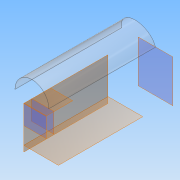
# Autodesk Inventor part: Top_Guard 1
Saved by Autodesk Inventor 2018.1 (Build 221171000, 171)
## iProperties
Created: 2019-03-23
Part Number: Top_Guard 1
Material: PMMA Plastic
Document SubType Name: Modeling
Designer: James
Density: 1.188 g/cm^3
Appearance: Polycarbonate - Clear
Author: James
Autodesk Inventor part; units mm, degrees
ref_plane "YZ Plane" through (0, 0, 0) normal (1, 0, 0) x (0, 1, 0)
ref_plane "XZ Plane" through (0, 0, 0) normal (0, 1, 0) x (-1, 0, 0)
ref_plane "XY Plane" through (0, 0, 0) normal (0, 0, 1) x (1, 0, 0)
derived "Top_Skeleton.ipt"
ref_plane "Work Plane1" through (0, 0, 0) normal (0, 0, 1) x (1, 0, 0)
ref_plane "Work Plane2" through (0, 0, 0) normal (0, 1, 0) x (-1, 0, 0)
ref_plane "Work Plane3" through (0, 0, 0) normal (1, 0, 0) x (0, 1, 0)
ref_plane "Work Plane4" through (0, 4100, 0) normal (0, 1, 0) x (-1, 0, 0)
ref_plane "Work Plane5" through (0, 0, -1300) normal (0, 0, 1) x (1, 0, 0)
ref_plane "Work Plane6" through (0, 275, 0) normal (0, 1, 0) x (-1, 0, 0)
sketch "Sketch1" plane through (0, 275, 0) normal (0, 1, 0) x (-1, 0, 0)
  arc A0 (610, 0) -> (-610, 0) centre (0, 0) ccw
  arc A1 (600, 0) -> (-600, 0) centre (0, 0) ccw
  line L0 (610, 0) -> (600, 0)
  line L1 (-600, 0) -> (-610, 0)
  dimension "d0" = 1200
  dimension "d1" = 10
  constraints: 4 end point, 4 point on circle, 2 centre point, 2 coincident, 2 horizontal alignment, 1 collinear, 1 horizontal
  measures "d0" diameter of A1
  measures "d1" radial gap between concentric circles of A0 A1
extrude "Extrusion1" add sketch "Sketch1" along normal up to surface (3825 mm away)
sketch "Sketch2" plane through (0, 0, 0) normal (1, 0, 0) x (0, 1, 0)
  line L0 (4100, 610) -> (4100, 0) projected
  line L1 (275, 0) -> (4100, 0) projected
  line L2 (4100, 0) -> (4100, 600) projected
  line L3 (4100, 0) -> (3896.5477, 1000)
  line L4 (3896.5477, 1000) -> (4100, 1000)
  line L5 (4100, 1000) -> (4100, 0)
  point P0 (0, 0)
  dimension "d6" = 11.5
  dimension "d7" = 1000
  constraints: 6 end point, 1 collinear, 1 perpendicular
  measures "d6" angle of L0 L3
  measures "d7" distance from line of L0.end L4
extrude "Extrusion2" cut sketch "Sketch2" along normal through all both and the other way through all
body "Solid1"
